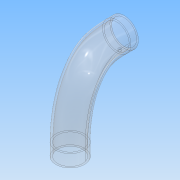
# Autodesk Inventor part: Top_Front Pipe 2
Saved by Autodesk Inventor 2018.1 (Build 221171000, 171)
## iProperties
Created: 2019-03-21
Part Number: Top_Front Pipe 2
Material: PMMA Plastic
Document SubType Name: Modeling
Designer: James
Density: 1.188 g/cm^3
Appearance: Polycarbonate - Clear
Author: James
Autodesk Inventor part; units mm, degrees
ref_plane "YZ Plane" through (0, 0, 0) normal (1, 0, 0) x (0, 1, 0)
ref_plane "XZ Plane" through (0, 0, 0) normal (0, 1, 0) x (-1, 0, 0)
ref_plane "XY Plane" through (0, 0, 0) normal (0, 0, 1) x (1, 0, 0)
sketch "Sketch1" plane through (0, 0, 0) normal (0, 1, 0) x (-1, 0, 0)
  circle A0 centre (0, 0) radius 23
  circle A1 centre (0, 0) radius 20
  dimension "d0" = 3
  dimension "d1" = 40
  constraints: 2 centre point, 2 coincident
  measures "d0" radial gap between concentric circles of A0 A1
  measures "d1" diameter of A1
extrude "Extrusion1" add sketch "Sketch1" along normal blind 12
sketch "Sketch2" plane through (0, 0, 0) normal (0, 0, 1) x (1, 0, 0)
  line L0 (23, 12) -> (-23, 12) projected
  point P0 (0, 0)
  point P1 (0, 5)
  point P2 (0, 12)
  dimension "d4" = 7
  constraints: 1 midpoint, 1 vertical alignment
  measures "d4" distance from line of L0 point (0, 5)
hole "Hole1" at (0, 5, 0) direction (0, 0, -1) diameter 4.5 end through all
sketch "Sketch3" plane through (0, 0, 0) normal (0, -1, 0) x (1, 0, 0)
  circle A0 centre (0, 0) radius 20 projected
  circle A1 centre (0, 0) radius 23 projected
sketch3d "3D Sketch1"
  spline S0 degree 4 poles (0, 0, 0) (0, -50, 0) (17.5, -50, 0) (17.5, -92.5, 0) (17.5, -92.5, -92.5) knots 1 1 1 1 1 2 2 2 2 2
  dimension "d12" = 50
  dimension "d14" = 42.5
  dimension "d15" = 92.5
  dimension "d20" = 17.5
sweep "Sweep1" add profiles "Sketch3" path "3D Sketch1"
sketch "Sketch4" plane through (17.5, -92.5, -92.5) normal (0, 0, -1) x (-1, 0, 0)
  spline S0 degree 6 poles (-19.4195, 4.7838) (-11.4711, 37.05) (29.5684, 31.8545) (53.3864, -13.1511) (11.3891, -41.9439) (-27.3679, -27.4825) (-19.4195, 4.7838) knots 0 0 0 0 0 0 0 1 1 1 1 1 1 1 weights 1.669078 1.03673 1.038347 0.853534 1.038347 1.03673 1.669078 projected
  circle A0 centre (0, 0) radius 23 projected
  point P0 (17.5, 92.5)
  point P1 (-22.3329, 5.4992)
  constraints: 2 other
extrude "Extrusion2" add sketch "Sketch4" along normal blind 20 contours S0 picked at (-20.1668, 8.4353)
body "Solid1"
